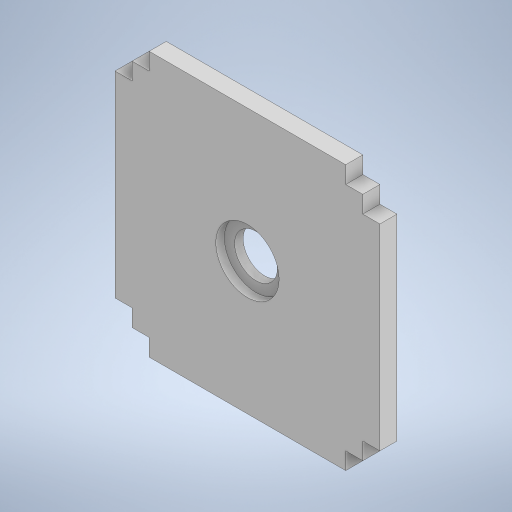
# Autodesk Inventor part: base
Saved by Autodesk Inventor 2023 (Build 270158000, 158)
## iProperties
Created: 2023-05-27
Part Number: base
Material: 一般
Document SubType Name: Modeling
Designer: 310611102
Density: 1 g/cm^3
Appearance: 預設
Author: 310611102
Autodesk Inventor part; units mm, degrees
ref_plane "YZ Plane" through (0, 0, 0) normal (1, 0, 0) x (0, 1, 0)
ref_plane "XZ Plane" through (0, 0, 0) normal (0, 1, 0) x (-1, 0, 0)
ref_plane "XY Plane" through (0, 0, 0) normal (0, 0, 1) x (1, 0, 0)
sketch "Sketch1" plane through (0, 0, 0) normal (0, 0, 1) x (1, 0, 0)
  line L0 (-57.5, 77.5) -> (57.5, 77.5)
  line L1 (77.5, 57.5) -> (77.5, -57.5)
  line L2 (57.5, -77.5) -> (-57.5, -77.5)
  line L3 (-77.5, -57.5) -> (-77.5, 57.5)
  line L4 (-50.6308, 50.6308) -> (50.6308, -50.6308) construction
  line L5 (50, 50) -> (-50, -50) construction
  line L6 (-40, 40) -> (-50.6308, 50.6308) construction
  line L7 (-57.5, 77.5) -> (-57.5, 67.5)
  line L8 (-57.5, 67.5) -> (-67.5, 67.5)
  line L9 (-67.5, 67.5) -> (-67.5, 57.5)
  line L10 (-67.5, 57.5) -> (-77.5, 57.5)
  line L11 (-67.5, -57.5) -> (-67.5, -67.5)
  line L12 (-77.5, -57.5) -> (-67.5, -57.5)
  line L13 (-67.5, -67.5) -> (-57.5, -67.5)
  line L14 (-57.5, -67.5) -> (-57.5, -77.5)
  line L15 (-40, -40) -> (-50.6308, -50.6308) construction
  line L16 (57.5, -67.5) -> (67.5, -67.5)
  line L17 (57.5, -77.5) -> (57.5, -67.5)
  line L18 (67.5, -67.5) -> (67.5, -57.5)
  line L19 (67.5, -57.5) -> (77.5, -57.5)
  line L20 (40, -40) -> (50.6308, -50.6308) construction
  line L21 (67.5, 57.5) -> (67.5, 67.5)
  line L22 (77.5, 57.5) -> (67.5, 57.5)
  line L23 (67.5, 67.5) -> (57.5, 67.5)
  line L24 (57.5, 67.5) -> (57.5, 77.5)
  line L25 (40, 40) -> (50.6308, 50.6308) construction
  circle A0 centre (0, 0) radius 12.5
  point P0 (-45.3154, 45.3154)
  point P1 (-45.3154, -45.3154)
  point P2 (45.3154, -45.3154)
  point P3 (45.3154, 45.3154)
  dimension "d9" = 155
  dimension "d17" = 360
  dimension "d19" = 10
  dimension "d20" = 25
  constraints: 52 end point, 7 coincident, 7 perpendicular, 3 midpoint, 2 parallel, 1 centre point, 1 horizontal, 1 point on line, 1 vertical, 53 other
  measures "d9" distance between parallel lines of L2 L0
  measures "d19" distance of L0.start L7.end
  measures "d20" diameter of A0
extrude "Extrusion1" add sketch "Sketch1" along normal blind 10
sketch "Sketch2" plane through (0, 0, 10) normal (0, 0, 1) x (1, 0, 0)
  circle A0 centre (0, 0) radius 18.5
  dimension "d21" = 37
  constraints: 1 centre point, 1 coincident
  measures "d21" diameter of A0
extrude "Extrusion2" cut sketch "Sketch2" against normal blind 5
body "Solid1"
